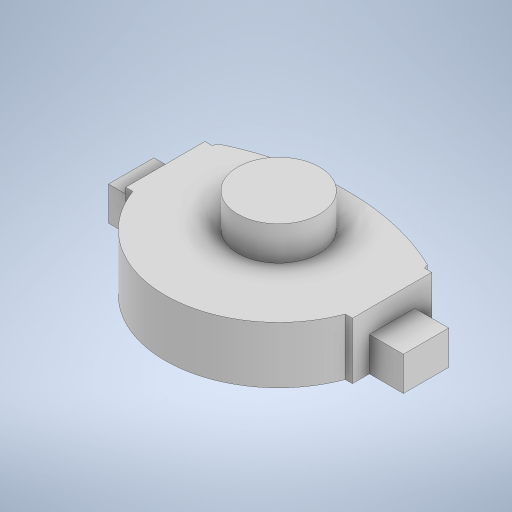
# Autodesk Inventor part: turntable
Saved by Autodesk Inventor 2024.3 (Build 283343000, 343)
## iProperties
Created: 2024-08-03
Part Number: turntable
Material: Generic
Document SubType Name: Modeling
Designer: compu
Density: 1 g/cm^3
Appearance: Default
Author: compu
Autodesk Inventor part; units mm, degrees
ref_plane "YZ Plane" through (0, 0, 0) normal (1, 0, 0) x (0, 1, 0)
ref_plane "XZ Plane" through (0, 0, 0) normal (0, 1, 0) x (-1, 0, 0)
ref_plane "XY Plane" through (0, 0, 0) normal (0, 0, 1) x (1, 0, 0)
sketch "Sketch1" plane through (0, 0, 0) normal (0, 1, 0) x (-1, 0, 0)
  circle A0 centre (0, 0) radius 10
  dimension "d0" = 20
  constraints: 1 centre point, 1 coincident
  measures "d0" diameter of A0
extrude "Extrusion1" add sketch "Sketch1" along normal blind 5
sketch "Sketch2" plane through (0, 5, 0) normal (0, 1, 0) x (1, 0, 0)
  line L0 (-14, 0) -> (14, 0) projected
  line L1 (0, 14) -> (0, -14) projected
  circle A0 centre (0, 0) radius 3.6
  dimension "d3" = 7.2
  constraints: 1 centre point, 1 coincident
  measures "d3" diameter of A0
extrude "Extrusion2" add sketch "Sketch2" along normal blind 3
sketch "Sketch3" plane through (0, 0, 0) normal (0, -1, 0) x (1, 0, 0)
  line L0 (10, -3.5) -> (-10, -3.5)
  line L1 (-10, -3.5) -> (-10, 3.5)
  line L2 (-10, 3.5) -> (10, 3.5)
  line L3 (10, 3.5) -> (10, -3.5)
  circle A0 centre (0, 0) radius 10 projected
  circle A1 centre (0, 0) radius 10 projected
  line L4 (-14, 0) -> (14, 0) projected
  line L5 (0, -14) -> (0, 14) projected
  line L6 (10, -2) -> (13, -2)
  line L7 (13, -2) -> (13, 2)
  line L8 (13, 2) -> (10, 2)
  line L9 (-10, -2) -> (-13, -2)
  line L10 (-13, -2) -> (-13, 2)
  line L11 (-13, 2) -> (-10, 2)
  dimension "d6" = 7
  dimension "d7" = 4
  dimension "d8" = 3
  dimension "d9" = 4
  dimension "d10" = 3
  constraints: 20 end point, 6 point on line, 5 perpendicular, 2 horizontal, 2 parallel, 2 tangent, 2 other
  measures "d6" distance between parallel lines of L2 L0
  measures "d7" distance of L6.end L7.end
  measures "d8" distance between parallel lines of L3 L7
  measures "d9" distance of L9.end L10.end
  measures "d10" distance between parallel lines of L1 L10
extrude "Extrusion3" add sketch "Sketch3" against normal up to surface (5 mm away) contours L0 A0 L3 | L0 L5 L4 A0 | L0 A0 L4 L5 | A0 L2 L3 | L4 L5 L2 A0 | L0 L1 A0 | L4 A0 L2 L5 | L1 L2 A0
extrude "Extrusion4" add sketch "Sketch3" against normal blind 3 contours L3 L4 L7 L6 | L3 L8 L7 L4 | L4 L10 L11 L1 | L1 L9 L10 L4
sketch "Sketch4" plane through (0, 0, 0) normal (0, -1, 0) x (1, 0, 0)
  arc A0 (9.3675, 3.5) -> (-9.3675, 3.5) centre (0, 0) ccw projected
  line L0 (-9.3675, 3.5) -> (-10, 3.5) projected
  line L1 (-10, 3.5) -> (-10, 2) projected
  line L2 (-10, 2) -> (-13, 2) projected
  line L3 (-13, 2) -> (-13, -2) projected
  line L4 (-13, -2) -> (-10, -2) projected
  line L5 (-10, -2) -> (-10, -3.5) projected
  line L6 (-10, -3.5) -> (-9.3675, -3.5) projected
  arc A1 (-9.3675, -3.5) -> (9.3675, -3.5) centre (0, 0) ccw projected
  line L7 (9.3675, -3.5) -> (10, -3.5) projected
  line L8 (10, -3.5) -> (10, -2) projected
  line L9 (10, -2) -> (13, -2) projected
  line L10 (13, -2) -> (13, 2) projected
  line L11 (13, 2) -> (10, 2) projected
  line L12 (10, 2) -> (10, 3.5) projected
  line L13 (10, 3.5) -> (9.3675, 3.5) projected
  line L14 (0, -31.9933) -> (0, 47.9155) projected
  line L15 (-29.75, 0) -> (29.75, 0) projected
  arc A2 (9.3675, 3.5) -> (-9.3675, 3.5) centre (0, 0) ccw projected
  circle A3 centre (0, 15.25) radius 21.25
  line L16 (15.0443, -6) -> (-18.096, -6) construction
  line L17 (10.2288, -3.7354) -> (10.2288, -20.5777)
  line L18 (10.2288, -20.5777) -> (-9.5456, -20.5777)
  line L19 (-9.5456, -20.5777) -> (-9.5456, -3.7354)
  line L20 (-9.5456, -3.7354) -> (-9.2762, -3.7354)
  line L21 (9.5456, -3.7354) -> (10.2288, -3.7354)
  dimension "d16" = 6
  constraints: 12 end point, 4 point on circle, 3 horizontal, 3 parallel, 2 perpendicular, 1 centre point, 1 point on line, 1 tangent
  measures "d16" distance between parallel lines of L15 L16
extrude "Extrusion5" cut sketch "Sketch4" against normal through all contours A3 A1 L14 | L14 A1 A3 | L14 L18 L19 A3 A1 | A1 A3 L21 L17 L18 L14
body "Solid1"
